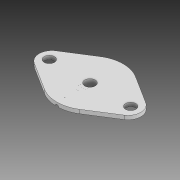
# Autodesk Inventor part: HD_rotor
Saved by Autodesk Inventor 2020 (Build 240168000, 168)
## iProperties
Created: 2021-03-19
Part Number: HD_rotor
Material: Generic
Document SubType Name: Modeling
Designer: DDeGo
Density: 1 g/cm^3
Appearance: Default
Author: DDeGo
Autodesk Inventor part; units mm, degrees
ref_plane "YZ Plane" through (0, 0, 0) normal (1, 0, 0) x (0, 1, 0)
ref_plane "XZ Plane" through (0, 0, 0) normal (0, 1, 0) x (-1, 0, 0)
ref_plane "XY Plane" through (0, 0, 0) normal (0, 0, 1) x (1, 0, 0)
sketch "608 bearing" plane through (0, 0, 0) normal (0, 0, 1) x (1, 0, 0)
  line L0 (-83.9037, 39.6189) -> (-76.9037, 39.6189) construction
  line L1 (-61.9037, 39.6189) -> (-61.9037, 32.6189) construction
  line L2 (-61.9037, 32.6189) -> (-68.9037, 32.6189) construction
  line L3 (-83.9037, 32.6189) -> (-83.9037, 39.6189) construction
  line L4 (-76.9037, 39.6189) -> (-76.9037, 32.6189) construction
  line L5 (-68.9037, 39.6189) -> (-68.9037, 32.6189) construction
  line L6 (-68.9037, 39.6189) -> (-61.9037, 39.6189) construction
  line L7 (-76.9037, 39.6189) -> (-68.9037, 39.6189) construction
  line L8 (-76.9037, 32.6189) -> (-83.9037, 32.6189) construction
  line L9 (-68.9037, 32.6189) -> (-76.9037, 32.6189) construction
  point P0 (-72.9037, 36.1189)
  point P1 (-72.9037, 39.6189)
  point P2 (-72.9037, 32.6189)
  dimension "d24" = 7
  dimension "d25" = 22
  dimension "d26" = 8
  measures "d24" distance of L1.start L1.end
  measures "d25" distance between parallel lines of L1 L3
  measures "d26" distance between parallel lines of L5 L4
derived "HD_mastersketch.ipt"
sketch "Belt" plane through (0, 0, 0) normal (0, 0, 1) x (1, 0, 0)
  line L0 (-44.56, 7.5) -> (-42.91, 7.5)
  line L1 (-42.91, 7.5) -> (-42.91, -7.5)
  line L2 (-42.91, -7.5) -> (-44.56, -7.5)
  line L3 (-44.56, -7.5) -> (-44.56, 7.5)
  point P0 (0, 0)
  point P1 (-44.56, 0)
sketch "Rotor" plane through (0, 0, 0) normal (0, 0, 1) x (1, 0, 0)
  line L0 (0, 0) -> (0, -29.5)
  line L1 (0, -29.5) -> (-4.075, -29.5)
  line L2 (-4.075, -29.5) -> (-4.075, -4.5)
  line L3 (-21.1933, -1.5) -> (-40.91, -1.5)
  line L4 (-40.91, -1.5) -> (-40.91, 1.5)
  line L5 (-40.91, 1.5) -> (-19.86, 1.5)
  line L6 (-4.075, 1.5) -> (-4.075, -4.5)
  line L7 (-4.075, 1.5) -> (-4.075, 13.5)
  line L8 (-4.075, 13.5) -> (0, 13.5)
  line L9 (0, 13.5) -> (0, 0)
  line L10 (-42.91, 7.5) -> (-42.91, -7.5) construction
  line L11 (-42.91, 0) -> (-40.91, 0) construction
  line L12 (-31.86, -2) -> (-31.86, -1.5) construction
  line L13 (-31.86, -1.5) -> (-31.86, 1.5) construction
  line L14 (-31.86, 2) -> (-31.86, 1.5) construction
  line L15 (-35.91, 1.5) -> (-35.91, -1.5) construction
  line L16 (-27.81, -1.5) -> (-27.81, 1.5) construction
  line L17 (-19.86, 1.5) -> (-19.86, -1.5) construction
  line L18 (-18.7933, -2.3) -> (-15.86, -4.5)
  line L19 (-15.86, -4.5) -> (-4.075, -4.5)
  line L20 (-19.86, 1.5) -> (-15.86, 1.5)
  line L21 (-15.86, 1.5) -> (-15.86, -4.5) construction
  line L22 (-15.86, 1.5) -> (-4.075, 1.5)
  line L23 (-35.91, 0) -> (-31.86, 0) construction
  line L24 (-31.86, 0) -> (-27.81, 0) construction
  arc A0 (-18.7933, -2.3) -> (-21.1933, -1.5) centre (-21.1933, -5.5) ccw
  line L25 (-42.86, 9) -> (-35.86, 9) construction
  line L26 (-20.86, 9) -> (-20.86, 2) construction
  line L27 (-20.86, 2) -> (-27.86, 2) construction
  line L28 (-42.86, 2) -> (-42.86, 9) construction
  line L29 (-35.86, 9) -> (-35.86, 2) construction
  line L30 (-27.86, 9) -> (-27.86, 2) construction
  line L31 (-27.86, 9) -> (-20.86, 9) construction
  line L32 (-35.86, 9) -> (-27.86, 9) construction
  line L33 (-35.86, 2) -> (-42.86, 2) construction
  line L34 (-27.86, 2) -> (-35.86, 2) construction
  line L35 (-42.86, -2) -> (-35.86, -2) construction
  line L36 (-20.86, -2) -> (-20.86, -9) construction
  line L37 (-20.86, -9) -> (-27.86, -9) construction
  line L38 (-42.86, -9) -> (-42.86, -2) construction
  line L39 (-35.86, -2) -> (-35.86, -9) construction
  line L40 (-27.86, -2) -> (-27.86, -9) construction
  line L41 (-27.86, -2) -> (-20.86, -2) construction
  line L42 (-35.86, -2) -> (-27.86, -2) construction
  line L43 (-35.86, -9) -> (-42.86, -9) construction
  line L44 (-27.86, -9) -> (-35.86, -9) construction
sketch "Base" plane through (0, 0, 0) normal (0, 0, 1) x (1, 0, 0)
  line L0 (0, -15.5) -> (-11.1, -15.5) construction
  line L1 (-52, -14.5) -> (-52, -1.25)
  line L2 (-51, -0.25) -> (-44.66, -0.25)
  line L3 (-37.86, -11.5) -> (-25.86, -11.5)
  line L4 (-19.86, -10) -> (-16.1, -5.5)
  line L5 (-16.1, -5.5) -> (-10.1, -5.5)
  line L6 (-10.1, -5.5) -> (-10.1, -7)
  line L7 (-10.1, -7) -> (-11.1, -8)
  line L8 (-11.1, -8) -> (-11.1, -15.5)
  line L9 (-11.1, -15.5) -> (-51, -15.5)
  line L10 (0, -15.5) -> (0, 38.4357) construction
  line L11 (-44.66, -0.25) -> (-44.66, -8)
  line L12 (-44.66, -8) -> (-42.66, -10)
  line L13 (-37.86, -10) -> (-37.86, -11.5)
  line L14 (-51, -0.25) -> (-52, -1.25)
  line L15 (-52, -14.5) -> (-51, -15.5)
  line L16 (-25.86, -11.5) -> (-25.86, -10)
  line L17 (-25.86, -10) -> (-19.86, -10)
  line L18 (-42.66, -10) -> (-37.86, -10)
  line L19 (0, 0) -> (-64.9444, 0) construction
  line L20 (-25.86, 11.5) -> (-25.86, 10)
  line L21 (-25.86, 10) -> (-19.86, 10)
  line L22 (-19.86, 10) -> (-16.1, 2.5)
  line L23 (-16.1, 2.5) -> (-10.1, 2.5)
  line L24 (-11.1, 5.5) -> (-11.1, 13)
  line L25 (-10.1, 2.5) -> (-10.1, 4.5)
  line L26 (-10.1, 4.5) -> (-11.1, 5.5)
  line L27 (0.103, 13) -> (-11.1, 13) construction
  line L28 (-37.86, 11.5) -> (-25.86, 11.5)
  line L29 (-11.1, 13) -> (-48.925, 13)
  line L30 (-49.925, 12) -> (-49.925, 1.25)
  line L31 (-48.925, 0.25) -> (-44.66, 0.25)
  line L32 (-37.86, 10) -> (-37.86, 11.5)
  line L33 (-42.66, 10) -> (-37.86, 10)
  line L34 (-44.66, 8) -> (-42.66, 10)
  line L35 (-44.66, 0.25) -> (-44.66, 8)
  line L36 (-49.925, 12) -> (-48.925, 13)
  line L37 (-48.925, 0.25) -> (-49.925, 1.25)
  line L38 (-44.56, -7.5) -> (-44.56, 7.5) construction
  line L39 (-42.91, -7.5) -> (-44.56, -7.5) construction
  line L40 (-31.86, -9) -> (-31.86, -11.5) construction
  line L41 (-40, 13) -> (-40, 12) construction
  line L42 (-40, 12) -> (-40, 10) construction
  line L43 (-40.26, -15.5) -> (-40.26, -12) construction
  line L44 (-40.26, -12) -> (-40.26, -10) construction
  line L45 (-35.86, -9) -> (-42.86, -9) construction
  line L46 (-15.86, -4.5) -> (-4.075, -4.5)
  line L47 (-15.86, 1.5) -> (-4.075, 1.5)
  line L48 (-11.1, 5.5) -> (-11.1, -8) construction
  point P0 (-52, -15.5)
  point P1 (-52, -0.25)
  point P2 (-49.925, 13)
  point P3 (-49.925, 0.25)
  point P4 (-31.86, 11.5)
revolve "Revolution1" add sketch "Rotor" angle 360 about axis through (0, 13.5, 0) along (0, -1, 0) contours L19 L18 A0 L3 L4 L5 L20 L22 L6
sketch "Sketch8" plane through (0, 1.5, 0) normal (0, 1, 0) x (1, 0, 0)
  circle A0 centre (0, 0) radius 40.91 projected
  line L0 (-40.6033, -5) -> (-13.8362, -21.9063)
  line L1 (-40.6033, -5) -> (-40.6033, 5) construction
  line L2 (-40.6033, 5) -> (-13.8362, 21.9063)
  circle A1 centre (0, 0) radius 4 construction
  line L3 (13.8362, -21.9063) -> (40.6033, -5)
  line L4 (40.6033, -5) -> (40.6033, 5) construction
  line L5 (40.6033, 5) -> (13.8362, 21.9063)
  arc A2 (-13.8362, -21.9063) -> (13.8362, -21.9063) centre (0, 0) ccw
  arc A3 (13.8362, 21.9063) -> (-13.8362, 21.9063) centre (0, 0) ccw
  dimension "d4" = 10
  dimension "d5" = 15
  constraints: 12 end point, 8 point on circle, 3 equal length, 2 centre point, 2 tangent, 2 vertical, 1 coincident, 1 concentric
  measures "d4" distance of L0.start L1.end
  measures "d5" radial gap between concentric circles of A0 A2
extrude "Extrusion1" cut sketch "Sketch8" against normal through all contours L5 A3 L2 A0 | A0 L0 A2 L3
sketch "Sketch9" plane through (0, 1.5, 0) normal (0, 1, 0) x (1, 0, 0)
  circle A0 centre (-31.86, 0) radius 4
  circle A1 centre (31.86, 0) radius 4
  circle A2 centre (0, 0) radius 16.1459 projected
  circle A3 centre (0, 0) radius 4.075 projected
  line L0 (0, 0) -> (0, 28.0271) construction
  point P0 (-35.86, 0)
  constraints: 2 end point, 1 centre point, 1 coincident, 1 horizontal alignment, 1 vertical, 3 other
extrude "Extrusion2" cut sketch "Sketch9" against normal through all contours A0 | A1
fillet "Fillet1" radius 10 4 edges at (40.6033, 0, 5) (40.6033, 0, -5) (-40.6033, 0, -5) (-40.6033, 0, 5)
sketch "Sketch10" plane through (0, -4.5, 0) normal (0, 1, 0) x (1, 0, 0)
  line L0 (-2.9, -6.2) -> (2.9, -6.2)
  line L1 (2.9, -6.2) -> (2.9, -3.7)
  line L2 (2.9, -3.7) -> (-2.9, -3.7)
  line L3 (-2.9, -3.7) -> (-2.9, -6.2)
  line L4 (-2.9, -6.2) -> (2.9, -3.7) construction
  line L5 (2.9, -6.2) -> (-2.9, -3.7) construction
  line L6 (0, 0) -> (0, -4.95) construction
  dimension "d11" = 3.7
  dimension "d12" = 2.5
  dimension "d13" = 5.8
  constraints: 14 end point, 2 midpoint, 2 parallel, 1 horizontal, 1 perpendicular, 1 vertical
  measures "d11" distance from line of L6.start L2
  measures "d12" distance of L0.end L1.end
  measures "d13" distance of L0.start L0.end
extrude "Extrusion3" cut sketch "Sketch10" along normal blind 5.8
sketch "Sketch14" plane through (0, 0, 0) normal (1, 0, 0) x (0, 1, 0)
  line L0 (-1.6, 6.2) -> (-1.6, 28.5259)
  line L1 (-1.6, 6.2) -> (0.05, 6.2)
  line L2 (0.05, 6.2) -> (0.05, 9.7)
  line L3 (0.05, 9.7) -> (1.4, 9.7)
  line L4 (1.4, 9.7) -> (1.4, 19.7)
  line L5 (1.4, 19.7) -> (-0.1, 19.7)
  line L6 (-0.1, 19.7) -> (-0.1, 28.5259)
  line L7 (-0.1, 28.5259) -> (-1.6, 28.5259)
  line L8 (-4.5, 6.2) -> (1.3, 6.2) projected
  point P0 (0, 0)
  point P1 (1.5, 0)
  dimension "d29" = 1.65
  dimension "d30" = 3
  dimension "d32" = 10
  dimension "d33" = 1.5
  dimension "d36" = 3.5
  constraints: 16 end point, 5 perpendicular, 2 vertical, 1 horizontal, 1 midpoint
  measures "d29" distance between parallel lines of L0 L2
  measures "d30" distance between parallel lines of L0 L4
  measures "d32" distance of L3.end L4.end
  measures "d33" distance between parallel lines of L0 L6
  measures "d36" distance between parallel lines of L8 L3
revolve "Revolution2" cut sketch "Sketch14" angle 360 about axis through (0, -1.6, 6.2) along (0, 0, 1)
fillet "Fillet3" radius 2 4 edges at (2.9793, -1.9515, 19.1164) (2.3432, -3.4733, 17.0688) (-2.9793, -1.9515, 19.1164) (-2.3428, -3.4738, 17.0682)
body "Solid1"
